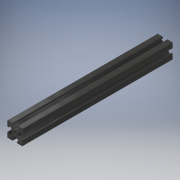
# Autodesk Inventor part: Beam_10mm
Saved by Autodesk Inventor 2019 (Build 230136000, 136)
## iProperties
Created: 2018-10-23
Part Number: Beam_10mm
Material: Generic
Document SubType Name: Modeling
Designer: xwermter
Density: 1 g/cm^3
Appearance: Default
Author: xwermter
Autodesk Inventor part; units mm, degrees
ref_plane "YZ Plane" through (0, 0, 0) normal (1, 0, 0) x (0, 1, 0)
ref_plane "XZ Plane" through (0, 0, 0) normal (0, 1, 0) x (-1, 0, 0)
ref_plane "XY Plane" through (0, 0, 0) normal (0, 0, 1) x (1, 0, 0)
sketch "Sketch1" plane through (0, 0, 0) normal (0, 0, 1) x (1, 0, 0)
  circle A0 centre (0, 0) radius 1.25
  line L0 (0, -7) -> (0, 7) projected
  line L1 (-7.0223, 0) -> (7.1337, 0) projected
  line L2 (5, 5) -> (1.5, 5)
  line L3 (1.5, 5) -> (1.5, 4)
  line L4 (5, 5) -> (5, 1.5)
  line L5 (-1, 2) -> (1, 2)
  line L6 (2, 1) -> (2, -1)
  line L7 (1, -2) -> (-1, -2)
  line L8 (-2, -1) -> (-2, 1)
  line L9 (1, 2) -> (3.3835, 4)
  line L10 (2, 2) -> (4.1114, 2) construction
  line L11 (3.3835, 4) -> (1.5, 4)
  line L12 (2, 1) -> (4, 3.3835)
  line L13 (2, 1) -> (5.1114, 1) construction
  line L14 (5, 1.5) -> (4, 1.5)
  line L15 (4, 1.5) -> (4, 3.3835)
  line L16 (5, 5) -> (5, 1.5)
  line L17 (-5, 5) -> (-1.5, 5)
  line L18 (1.5, 5) -> (5, 5)
  line L19 (5, 5) -> (5, 1.5)
  line L20 (5, 0) -> (5, -5)
  line L21 (-2, 1) -> (-4, 3.3835)
  line L22 (-4, 3.3835) -> (-4, 1.5)
  line L23 (-5, 1.5) -> (-4, 1.5)
  line L24 (-5, 5) -> (-5, 1.5)
  line L25 (-5, 5) -> (-1.5, 5)
  line L26 (-1.5, 5) -> (-1.5, 4)
  line L27 (-1.5, 4) -> (-3.3835, 4)
  line L28 (-1, 2) -> (-3.3835, 4)
  line L29 (-1, -2) -> (-3.3835, -4)
  line L30 (-3.3835, -4) -> (-1.5, -4)
  line L31 (-1.5, -5) -> (-1.5, -4)
  line L32 (-5, -5) -> (-1.5, -5)
  line L33 (-5, -5) -> (-5, -1.5)
  line L34 (-5, -1.5) -> (-4, -1.5)
  line L35 (-4, -1.5) -> (-4, -3.3835)
  line L36 (-2, -1) -> (-4, -3.3835)
  line L37 (2, -1) -> (4, -3.3835)
  line L38 (4, -3.3835) -> (4, -1.5)
  line L39 (5, -1.5) -> (4, -1.5)
  line L40 (5, -5) -> (5, -1.5)
  line L41 (5, -5) -> (1.5, -5)
  line L42 (1.5, -5) -> (1.5, -4)
  line L43 (1.5, -4) -> (3.3835, -4)
  line L44 (1, -2) -> (3.3835, -4)
  line L45 (-5, -5) -> (-5, -1.5)
  line L46 (-5, 1.5) -> (-5, 5)
  line L47 (5, -5) -> (1.5, -5)
  line L48 (-1.5, -5) -> (-5, -5)
  dimension "d0" = 2.5
  dimension "d3" = 3.5
  dimension "d4" = 1
  dimension "d5" = 90
  dimension "d6" = 3.5
  dimension "d10" = 2
  dimension "d11" = 40
  dimension "d13" = 50
  dimension "d14" = 1
  dimension "d17" = 360
  dimension "d19" = 3.1115
  constraints: 94 end point, 10 parallel, 8 perpendicular, 6 horizontal, 6 point on line, 2 coincident, 2 symmetric about line, 1 centre point, 1 collinear, 1 equal length, 74 other
  measures "d0" diameter of A0
  measures "d3" distance of L2.start L2.end
  measures "d4" distance of L2.end L3.end
  measures "d5" angle of L3 L2
  measures "d6" distance of L2.start L4.end
  measures "d10" distance of L5.start L5.end
  measures "d11" angle of L10 L9
  measures "d13" angle of L13 L12
  measures "d14" distance of L4.end L14.end
  measures "d19" distance of L5.end L9.end
extrude "Extrusion1" add sketch "Sketch1" along normal mid plane 100 contours L1 L6 L37 L38 L39 L20 L41 L42 L43 L44 L7 L0 A0 | A0 L0 L5 L9 L11 L3 L2 L4 L14 L15 L12 L6 L1 | A0 L1 L8 L21 L22 L23 L24 L17 L26 L27 L28 L5 L0 | L0 L7 L29 L30 L31 L32 L33 L34 L35 L36 L8 L1 A0
fillet "Fillet1" radius 0.18 28 edges at (-5, 5, 0) (-5, 1.5, 0) (-1.5, 5, 0) (-1.5, 4, 0) (-4, 1.5, 0) (-3.3835, 4, 0) (-4, 3.3835, 0) (1.5, 5, 0) (5, 5, 0) (3.3835, 4, 0) (4, 3.3835, 0) (4, 1.5, 0) (5, 1.5, 0) (1.5, 4, 0) (4, -1.5, 0) (5, -1.5, 0) (5, -5, 0) (4, -3.3835, 0) (3.3835, -4, 0) (1.5, -4, 0) (1.5, -5, 0) (-3.3835, -4, 0) (-4, -3.3835, 0) (-4, -1.5, 0) (-5, -1.5, 0) (-5, -5, 0) (-1.5, -5, 0) (-1.5, -4, 0)
fillet "Fillet2" radius 0.3 8 edges at (-1, 2, 0) (1, 2, 0) (2, -1, 0) (2, 1, 0) (1, -2, 0) (-1, -2, 0) (-2, -1, 0) (-2, 1, 0)
thread "Thread1" size "M3x0.5" class "6H" standard "ANSI Metric M Profile" length 8
thread "Thread2" size "M3x0.5" class "6H" standard "ANSI Metric M Profile" length 8
body "Solid1"
